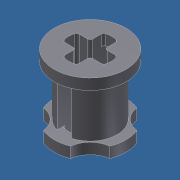
# Autodesk Inventor part: 3713
Saved by Autodesk Inventor 2011 SP2 (Build 150553200, 553)
## iProperties
Company: Allseas Engineering BV
Created: 2011-11-29
Part Number: 3713
Cost Center: 0 kg
Material: Steel
Document SubType Name: Modeling
Designer: PMe
Authority: 0 mm^3
Stock Number: =<Filenr>_<Document number>
Mass: 1.25037 g
Surface Area: 3.92738 cm^2
Volume: 0.159283 cm^3
Density: 7.85 g/cm^3
Act. Code: DW000
SaveDate: 2011-07-28
SaveTime: 18:32
FileName: Standard
TotalMass: 0 kg
TotalVolume: 0 mm^3
Subject: =<Title><TITLE 1_2> <TITLE 2_2>
Author: PMe
Autodesk Inventor part; units mm, degrees
ref_plane "YZ Plane" through (0, 0, 0) normal (1, 0, 0) x (0, 1, 0)
ref_plane "XZ Plane" through (0, 0, 0) normal (0, 1, 0) x (-1, 0, 0)
sketch "Sketch1" plane through (0, 0, 0) normal (0, 0, 1) x (1, 0, 0)
  circle A0 centre (0, 0) radius 4
  dimension "d0" = 8
  constraints: 1 centre point, 1 coincident
  measures "d0" diameter of A0
extrude "Extrusion1" add sketch "Sketch1" along normal mid plane 8
sketch "Sketch2" plane through (0, 0, 4) normal (0, 0, 1) x (1, 0, 0)
  circle A0 centre (0, 0) radius 2.4
  line L0 (-2.2627, 0.8) -> (-0.8, 0.8)
  line L1 (-0.8, 0.8) -> (-0.8, 2.2627)
  line L2 (0.8, 2.2627) -> (0.8, 0.8)
  line L3 (0.8, 0.8) -> (2.2627, 0.8)
  line L4 (2.2627, -0.8) -> (0.8, -0.8)
  line L5 (0.8, -0.8) -> (0.8, -2.2627)
  line L6 (-0.8, -2.2627) -> (-0.8, -0.8)
  line L7 (-0.8, -0.8) -> (-2.2627, -0.8)
  dimension "d3" = 4.8
  dimension "d4" = 1.6
  constraints: 16 end point, 7 equal length, 5 perpendicular, 2 parallel, 1 coincident, 1 horizontal, 10 other
  measures "d4" distance between parallel lines of L5 L6
extrude "Extrusion2" cut sketch "Sketch2" against normal through all contours A0 L4 L5 L6 L7 L0 L1 L2 L3
ref_plane "Work Plane1" through (0, 0, -2.8) normal (0, 0, -1) x (-1, 0, 0)
sketch "Sketch3" plane through (0, 0, -2.8) normal (0, 0, -1) x (-1, 0, 0)
  circle A0 centre (0, 0) radius 4 projected
  circle A1 centre (0, 0) radius 4 projected
  circle A2 centre (0, 0) radius 3
  dimension "d8" = 6
  constraints: 1 centre point, 1 coincident
  measures "d8" diameter of A2
extrude "Extrusion3" cut sketch "Sketch3" against normal blind 5.6
sketch "Sketch4" plane through (0, 0, -4) normal (0, 0, -1) x (-1, 0, 0)
  circle A0 centre (4, -4) radius 2.5
  point P0 (0, 0)
  dimension "d11" = 4
  dimension "d12" = 4
  dimension "d13" = 5
  constraints: 1 centre point
  measures "d11" horizontal distance of A0.centre point (0, 0)
  measures "d12" horizontal distance of point (0, 0) A0.centre
  measures "d13" diameter of A0
extrude "Extrusion4" cut sketch "Sketch4" against normal up to surface (1.2 mm away)
pattern_circular "Circular Pattern1" count 4 over 360 about axis through (0, 0, -10) along (0, 0, 1) of "Extrusion4"
sketch "Sketch5" plane through (0, 0, 0) normal (0, 1, 0) x (-1, 0, 0)
  line L0 (-0.8, 4) -> (-0.8, -4) projected
  line L1 (0.8, 4) -> (0.8, -4) projected
  line L2 (4, 2.8) -> (-4, 2.8) projected
  line L3 (-1.518, -2.8) -> (1.518, -2.8) projected
  line L4 (-0.8, -2.8) -> (0.8, -2.8)
  line L5 (0.8, -2.8) -> (0.8, 2.8)
  line L6 (0.8, 2.8) -> (-0.8, 2.8)
  line L7 (-0.8, 2.8) -> (-0.8, -2.8)
  point P0 (0, 0)
  constraints: 8 end point, 4 point on line, 2 parallel, 1 horizontal, 1 perpendicular
extrude "Extrusion5" cut sketch "Sketch5" along normal through all both and the other way through all
fillet "Fillet1" radius 0.3 16 edges at (-0.8, 0.8, 0) (-0.8, -0.8, 0) (0.8, -0.8, 0) (0.8, 0.8, 0) (-2.2627, -0.8, 0) (-2.2627, 0.8, 0) (-0.8, 2.2627, 3.4) (0.8, 2.2627, 3.4) (2.2627, 0.8, 0) (2.2627, -0.8, 0) (0.8, -2.2627, 3.4) (-0.8, -2.2627, 3.4) (0.8, 2.2627, -3.4) (-0.8, 2.2627, -3.4) (0.8, -2.2627, -3.4) (-0.8, -2.2627, -3.4)
body "Solid1"
